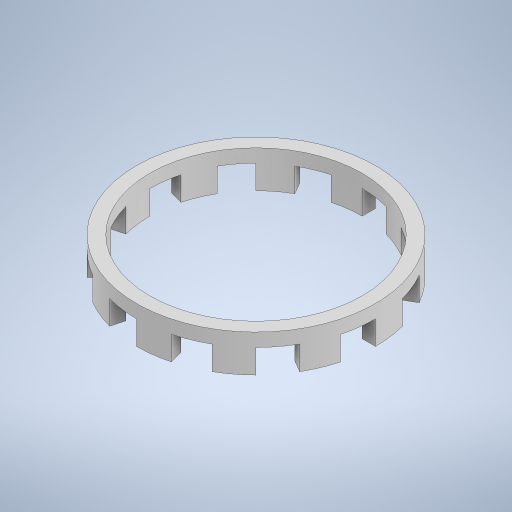
# Autodesk Inventor part: 4 Castle Spacer
Saved by Autodesk Inventor 2024 (Build 280153000, 153)
## iProperties
Created: 2024-04-17
Part Number: 4 Castle Spacer
Material: Generic
Document SubType Name: Modeling
Designer: Tommy Rohmann
Density: 1 g/cm^3
Appearance: Default
Author: Tommy Rohmann
Autodesk Inventor part; units mm, degrees
ref_plane "YZ Plane" through (0, 0, 0) normal (1, 0, 0) x (0, 1, 0)
ref_plane "XZ Plane" through (0, 0, 0) normal (0, 1, 0) x (-1, 0, 0)
ref_plane "XY Plane" through (0, 0, 0) normal (0, 0, 1) x (1, 0, 0)
sketch "Sketch1" plane through (0, 0, 0) normal (0, 1, 0) x (-1, 0, 0)
  circle A0 centre (0, 0) radius 57.15
  circle A1 centre (0, 0) radius 50.8
  line L0 (0, 0) -> (0, -57.15)
  line L1 (0, 0) -> (57.15, 0) construction
  line L2 (49.069, -13.148) -> (55.2027, -14.7915)
  line L3 (0, 0) -> (57.15, 0) construction
  line L4 (0, 0) -> (57.15, 0)
  line L5 (43.9941, -25.4) -> (49.4934, -28.575)
  line L6 (0, 0) -> (57.15, 0) construction
  line L7 (50.8, 0) -> (57.15, 0)
  line L8 (49.069, 13.148) -> (55.2027, 14.7915)
  line L9 (43.9941, 25.4) -> (49.4934, 28.575)
  line L10 (35.921, 35.921) -> (40.4112, 40.4112)
  line L11 (25.4, 43.9941) -> (28.575, 49.4934)
  line L12 (13.148, 49.069) -> (14.7915, 55.2027)
  line L13 (0, 50.8) -> (0, 57.15)
  line L14 (-13.148, 49.069) -> (-14.7915, 55.2027)
  line L15 (-25.4, 43.9941) -> (-28.575, 49.4934)
  line L16 (-35.921, 35.921) -> (-40.4112, 40.4112)
  line L17 (-43.9941, 25.4) -> (-49.4934, 28.575)
  line L18 (-49.069, 13.148) -> (-55.2027, 14.7915)
  line L19 (-50.8, 0) -> (-57.15, 0)
  line L20 (-49.069, -13.148) -> (-55.2027, -14.7915)
  line L21 (-43.9941, -25.4) -> (-49.4934, -28.575)
  line L22 (-35.921, -35.921) -> (-40.4112, -40.4112)
  line L23 (-25.4, -43.9941) -> (-28.575, -49.4934)
  line L24 (-13.148, -49.069) -> (-14.7915, -55.2027)
  line L25 (0, -50.8) -> (0, -57.15)
  line L26 (13.148, -49.069) -> (14.7915, -55.2027)
  line L27 (25.4, -43.9941) -> (28.575, -49.4934)
  line L28 (35.921, -35.921) -> (40.4112, -40.4112)
  point P0 (50.8, 0)
  point P1 (0, -50.8)
  dimension "d0" = 114.3
  dimension "d1" = 101.6
  dimension "d3" = 15
  dimension "d4" = 30
  dimension "d7" = 360
  constraints: 58 end point, 3 horizontal, 2 coincident, 1 collinear, 1 vertical, 84 other
  measures "d3" angle of L2 L3
  measures "d4" angle of L5 L6
extrude "Extrusion1" add sketch "Sketch1" along normal blind 6.35 contours L4 A1 L8 A0 | A0 L2 A1 L4 | L8 A1 L9 A0 | A0 L5 A1 L2 | L9 A1 L10 A0 | A0 L28 A1 L5 | L10 A1 L11 A0 | A0 L27 A1 L28 | L0 A0 L24 A1 | A1 L26 A0 L0 | L11 A1 L12 A0 | A0 L26 A1 L27 | L24 A0 L23 A1 | L12 A1 L13 A0 | L23 A0 L22 A1 | L13 A1 L14 A0 | L22 A0 L21 A1 | L14 A1 L15 A0 | L21 A0 L20 A1 | L15 A1 L16 A0 | L20 A0 L19 A1 | L16 A1 L17 A0 | L19 A0 L18 A1 | L17 A1 L18 A0
extrude "Extrusion2" add sketch "Sketch1" against normal blind 11.43 contours L4 A1 L8 A0 | A0 L5 A1 L2 | L9 A1 L10 A0 | A0 L27 A1 L28 | A1 L26 A0 L0 | L11 A1 L12 A0 | L24 A0 L23 A1 | L13 A1 L14 A0 | L22 A0 L21 A1 | L15 A1 L16 A0 | L20 A0 L19 A1 | L17 A1 L18 A0
body "Solid1"
